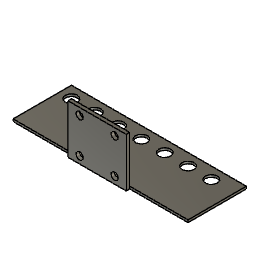
Tank Track Chassis v1 (Autodesk Fusion 360 design; units mm, degrees)
Autodesk Fusion 360 part; units mm, degrees
sketch "Sketch1" plane through (0, 0, 0) normal (0, 0, 1) x (1, 0, 0)
  line L0 (0, 0) -> (-150, 0)
  line L1 (-150, 0) -> (-150, -50)
  line L2 (-150, -50) -> (0, -50)
  line L3 (0, -50) -> (0, 0)
  dimension "d1" = 150
  constraint horizontal L0
  constraint vertical L1
  constraint horizontal L2
  constraint vertical L3
  constraint coincident L0.start L3.end
  measures "d1" distance of L0.start L0.end
extrude "Extrude1" add sketch "Sketch1" along normal blind 1
sketch "Sketch2" plane through (0, -50, 0) normal (0, -1, 0) x (1, 0, 0)
  line L0 (-150, 0) -> (0, 0)
  line L1 (0, 0) -> (0, 1)
  line L2 (0, 1) -> (-150, 1)
  line L3 (-150, 1) -> (-150, 0)
  line L4 (-100, 0) -> (-50, 0)
  line L5 (-50, 0) -> (-50, 1)
  line L6 (-50, 1) -> (-100, 1)
  line L7 (-100, 1) -> (-100, 0)
  dimension "d4" = 50
  constraint horizontal L4
  constraint vertical L5
  constraint horizontal L6
  constraint vertical L7
  constraint coincident L0 L4.start
  measures "d4" distance of L4.start L4.end
extrude "Extrude2" add sketch "Sketch2" along normal blind 1 contours L0 L2 L4 L5 L6 L7
extrude "Extrude3" add 1 faces at (-83.3333, -51, 0.6667) along direction (0, -1, 0) blind 2
sketch "Sketch3" plane through (0, 0, 1) normal (0, 0, 1) x (-1, 0, 0)
  line L0 (0, 50) -> (0, 0)
  line L1 (0, 0) -> (150, 0)
  line L2 (150, 0) -> (150, 50)
  line L3 (150, 50) -> (100, 50)
  line L4 (100, 50) -> (100, 53)
  line L5 (100, 53) -> (50, 53)
  line L6 (50, 53) -> (50, 50)
  line L7 (50, 50) -> (0, 50)
  line L8 (100, 50) -> (50, 50)
  line L9 (50, 50) -> (50, 53)
  line L10 (50, 53) -> (100, 53)
  line L11 (100, 53) -> (100, 50)
  constraint horizontal L8
  constraint vertical L9
  constraint horizontal L10
  constraint vertical L11
  constraint coincident L5.end L6.start
  constraint coincident L3.end L4.start
extrude "Extrude4" add sketch "Sketch3" along normal blind 40 contours L4 L5 L6 L8 L9 L10 L11
extrude "Extrude5" add 1 faces at (-83.3333, -16.6667, 0) along direction (0, 0, -1) blind 1
sketch "Sketch4" plane through (0, -53, 0) normal (0, -1, 0) x (1, 0, 0)
  line L0 (-100, 41) -> (-100, -1)
  line L1 (-100, -1) -> (-50, -1)
  line L2 (-50, -1) -> (-50, 41)
  line L3 (-50, 41) -> (-100, 41)
  circle A0 centre (-60, 35) radius 3
  circle A1 centre (-60, 5) radius 3
  dimension "d13" = 6
  dimension "d14" = 6
  measures "d13" diameter of A0
  measures "d14" diameter of A1
sketch "Sketch5" plane through (0, -53, 0) normal (0, -1, 0) x (1, 0, 0)
  circle A0 centre (-90, 35) radius 3
  circle A1 centre (-90, 5) radius 3
  dimension "d15" = 6
  dimension "d16" = 6
  measures "d15" diameter of A0
  measures "d16" diameter of A1
extrude "Extrude6" cut sketch "Sketch4" sketch "Sketch5" against normal blind 15 contours A0 | A1 of sketch 2
sketch "Sketch6" plane through (0, 0, -1) normal (0, 0, -1) x (1, 0, 0)
  line L0 (0, 0) -> (0, 50)
  line L1 (0, 50) -> (-50, 50)
  line L2 (-50, 50) -> (-50, 53)
  line L3 (-50, 53) -> (-100, 53)
  line L4 (-100, 53) -> (-100, 50)
  line L5 (-100, 50) -> (-150, 50)
  line L6 (-150, 50) -> (-150, 0)
  line L7 (-150, 0) -> (0, 0)
  circle A0 centre (-140, 10) radius 5.1
  circle A1 centre (-120, 10) radius 5.1
  circle A2 centre (-100, 10) radius 5.1
  circle A3 centre (-80, 10) radius 5.1
  circle A4 centre (-60, 10) radius 5.1
  circle A5 centre (-40, 10) radius 5.1
  circle A6 centre (-20, 10) radius 5.1
  dimension "d19" = 10.2
  dimension "d20" = 10.2
  dimension "d21" = 10.2
  dimension "d22" = 10.2
  dimension "d23" = 10.2
  dimension "d24" = 10.2
  dimension "d25" = 10.2
  measures "d19" diameter of A0
  measures "d20" diameter of A1
  measures "d21" diameter of A2
  measures "d22" diameter of A3
  measures "d23" diameter of A4
  measures "d24" diameter of A5
  measures "d25" diameter of A6
extrude "Extrude7" cut sketch "Sketch6" against normal blind 10 contours A0 | A1 | A2 | A3 | A4 | A5 | A6
